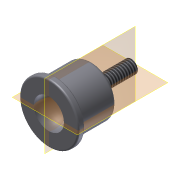
# Autodesk Inventor part: transfer_housing
Saved by Autodesk Inventor 2012 (Build 160160000, 160)
## iProperties
Created: 2011-01-09
Part Number: transfer_housing
Material: Steel
Document SubType Name: Modeling
Designer: Antonella Wilby
Mass: 72.1484 g
Surface Area: 24.3457 cm^2
Volume: 9.19088 cm^3
Density: 7.85 g/cm^3
Author: Antonella Wilby
Autodesk Inventor part; units mm, degrees
ref_plane "XY Plane" through (0, 0, 0) normal (0, 0, 1) x (1, 0, 0)
sketch "Sketch1" plane through (0, 0, 0) normal (0, 0, 1) x (1, 0, 0)
  circle A0 centre (0, 0) radius 14.2875
  dimension "d0" = 28.575
  constraints: 1 centre point, 1 coincident
  measures "d0" diameter of A0
extrude "Extrusion1" add sketch "Sketch1" along normal mid plane 20.6375
sketch "Sketch2" plane through (0, 0, -10.3188) normal (0, 0, -1) x (-1, 0, 0)
  circle A0 centre (0, 0) radius 14.2875 projected
  circle A1 centre (0, 0) radius 11.9062
  dimension "d3" = 23.8125
  constraints: 1 centre point, 1 coincident
  measures "d3" diameter of A1
extrude "Extrusion2" cut sketch "Sketch2" against normal blind 17.4625
sketch "Sketch3" plane through (0, 0, -10.3188) normal (0, 0, -1) x (-1, 0, 0)
  circle A0 centre (0, 0) radius 11.9062 projected
  circle A1 centre (0, 0) radius 3.175
  dimension "d6" = 6.35
  constraints: 1 centre point, 1 coincident
  measures "d6" diameter of A1
extrude "Extrusion3" add sketch "Sketch3" along normal blind 19.05 contours A1
thread "Thread1" size "1/4-20 UNC" class "2A" standard "ANSI Unified Screw Threads" full length
ref_plane "Work Plane1" through (0, 0, 7.1438) normal (0, 0, 1) x (1, 0, 0)
sketch "Sketch4" plane through (0, 0, 7.1438) normal (0, 0, 1) x (1, 0, 0)
  line L0 (-20.0025, 0) -> (20.0025, 0) projected
  line L1 (0, -20.0025) -> (0, 20.0025) projected
  arc A0 (0, -7.9375) -> (0, 7.9375) centre (0, 0) ccw
  line L2 (0, -7.9375) -> (0, 7.9375)
  dimension "d12" = 15.875
  constraints: 2 end point, 2 point on circle, 2 point on line, 1 centre point, 1 coincident
  measures "d12" diameter of A0
revolve "Revolution1" cut sketch "Sketch4" angle 360 about axis through (0, -10, 7.1438) along (0, 1, 0)
fillet "Fillet1" radius 1.5875 1 edges at (11.9062, 0, -10.3188)
fillet "Fillet2" radius 0.7937 1 edges at (-14.2875, 0, 7.1438)
fillet "Fillet3" radius 0.7937 1 edges at (-14.2875, 0, 10.3188)
body "Solid1"
